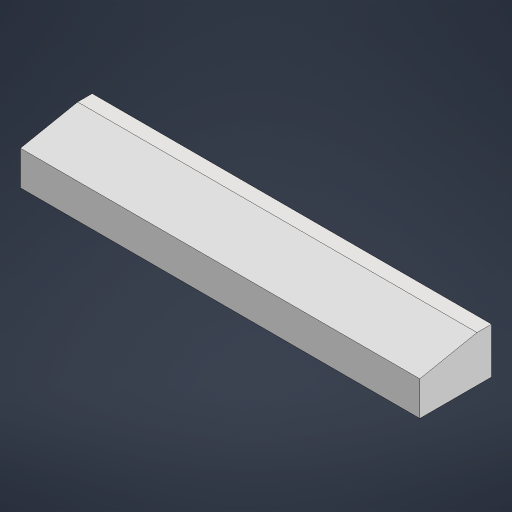
# Autodesk Inventor part: WDW_sill
Saved by Autodesk Inventor 2023.1 (Build 271208000, 208)
## iProperties
Created: 2022-11-19
Part Number: WDW_sill
Material: Generic
Document SubType Name: Modeling
Designer: awelt
Mass: 33595.5 g
Surface Area: 8915.83 cm^2
Volume: 33595.5 cm^3
Density: 1 g/cm^3
Appearance: Default
RuleStatus: InUse
BeforeDocSave0: file://C:\Users\awelt\Documents\Inventor\iLogic_Rules\BoundingStore
DocClose0: file://C:\Users\awelt\Documents\Inventor\iLogic_Rules\BoundingStore
Author: awelt
BoundingBL1: 5 1/2
BoundingBL2: 8 5/8
BoundingBL3: 48
BoundingCF: 1.318
Autodesk Inventor part; units mm, degrees
ref_plane "YZ Plane" through (0, 0, 0) normal (1, 0, 0) x (0, 1, 0)
ref_plane "XZ Plane" through (0, 0, 0) normal (0, 1, 0) x (-1, 0, 0)
ref_plane "XY Plane" through (0, 0, 0) normal (0, 0, 1) x (1, 0, 0)
sketch "Sketch2" plane through (0, 0, 0) normal (1, 0, 0) x (0, 1, 0)
  line L0 (0, 0) -> (0, 219.075)
  line L1 (0, 0) -> (139.7, 0)
  line L2 (139.7, 0) -> (139.7, 44.45)
  line L3 (139.7, 44.45) -> (104.775, 219.075)
  line L4 (104.775, 219.075) -> (0, 219.075)
  dimension "d3" = 219.075
  dimension "d4" = 139.7
  dimension "d5" = 44.45
  dimension "d6" = 34.925
  dimension "d7" = 104.775
  constraints: 10 end point, 2 perpendicular, 1 horizontal, 1 vertical
  measures "d3" distance of L0.start L0.end
  measures "d4" distance of L0.start L1.end
  measures "d5" distance of L1.end L2.end
  measures "d6" horizontal distance of L3.end L2.end
  measures "d7" distance of L3.end L0.end
extrude "Extrusion1" add sketch "Sketch2" along normal blind 1219.2
body "Solid1"
